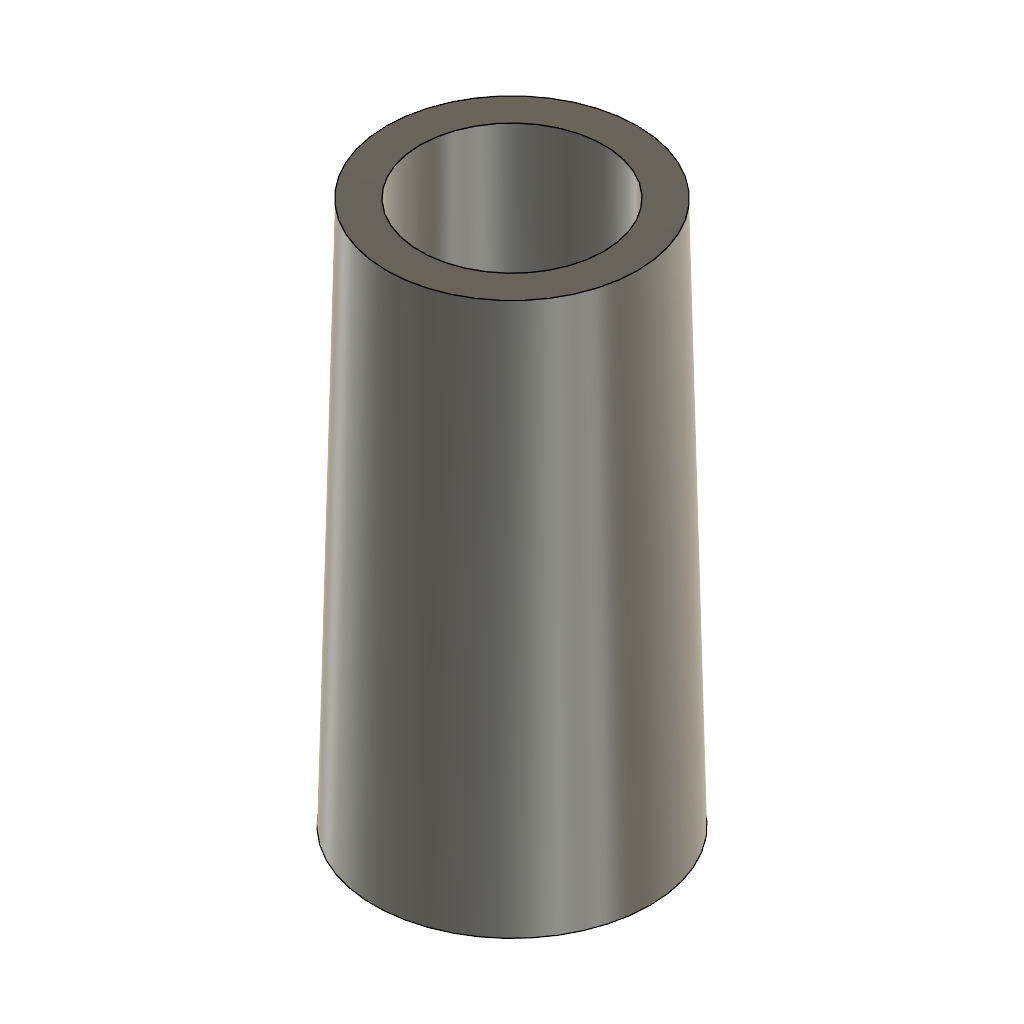
clarinet-barrel (Autodesk Fusion 360 design; units mm, degrees)
Autodesk Fusion 360 part; units mm, degrees
sketch "Sketch1" plane through (0, 0, 0) normal (0, 0, 1) x (1, 0, 0)
  circle A0 centre (0, 0) radius 16.5
  circle A1 centre (0, 0) radius 12
  circle A2 centre (0, 0) radius 6.5
  dimension "d1" = 33
  dimension "d2" = 24
  dimension "d3" = 13
  constraint coincident A0.centre A1.centre
  constraint concentric A0 A1
  constraint concentric A0 A2
  measures "d1" diameter of A0
  measures "d2" diameter of A1
  measures "d3" diameter of A2
ref_plane "WorkPlane1" through (0, 0, 65) normal (0, 0, 1) x (1, 0, 0)
sketch "Sketch2" plane through (0, 0, 65) normal (0, 0, 1) x (1, 0, 0)
  circle A0 centre (0, 0) radius 15
  circle A1 centre (0, 0) radius 11
  circle A2 centre (0, 0) radius 7
  dimension "d6" = 30
  dimension "d7" = 22
  dimension "d8" = 14
  constraint coincident A0.centre A1.centre
  measures "d6" diameter of A0
  measures "d7" diameter of A1
  measures "d8" diameter of A2
loft "Loft1" add profiles "Sketch1", "Sketch2" section 1 contours A0 section 2 contours A0
loft "Loft2" cut profiles "Sketch2", "Sketch1" section 1 contours A2 section 2 contours A2
extrude "Extrude1" cut sketch "Sketch2" against normal blind 19 contours A1
extrude "Extrude2" cut sketch "Sketch1" along normal blind 19 contours A1
delete_face "DeleteFace1" 1 faces at (6.9652, -0.697, 52.3333)
